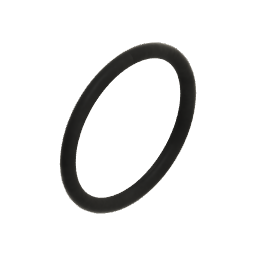
063d16ca-c277-448f-8e48-6c60c6a685a3 (Autodesk Fusion 360 design; units mm, degrees)
Autodesk Fusion 360 part; units mm, degrees
sketch "Esboço2" plane through (0, 0, 0) normal (0, 0, 1) x (1, 0, 0)
  line L0 (38, 70) -> (46, 70)
  circle A0 centre (38.0313, 86) radius 1.5
  dimension "d439" = 3
  dimension "d440" = 16
  constraint horizontal L0
  measures "d439" diameter of A0
  measures "d440" distance of L0 A0.centre
revolve "Revolucionar1" add sketch "Esboço2" angle 360 about axis through (38, 70, 0) along (1, 0, 0)
